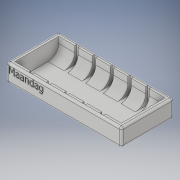
# Autodesk Inventor part: Maandag
Saved by Autodesk Inventor 2019 (Build 230136000, 136)
## iProperties
Created: 2020-10-20
Part Number: Maandag
Material: Generic
Document SubType Name: Modeling
Designer: daanswinters
Density: 1 g/cm^3
Appearance: Default
Author: daanswinters
Autodesk Inventor part; units mm, degrees
ref_plane "YZ Plane" through (0, 0, 0) normal (1, 0, 0) x (0, 1, 0)
ref_plane "XZ Plane" through (0, 0, 0) normal (0, 1, 0) x (-1, 0, 0)
ref_plane "XY Plane" through (0, 0, 0) normal (0, 0, 1) x (1, 0, 0)
sketch "Sketch1" plane through (0, 0, 0) normal (0, 0, 1) x (1, 0, 0)
  line L0 (55, -8.5) -> (-55, -8.5)
  line L1 (-55, -8.5) -> (-55, 8.5)
  line L2 (-55, 8.5) -> (55, 8.5)
  line L3 (55, 8.5) -> (55, -8.5)
  line L4 (55, -8.5) -> (-55, 8.5) construction
  line L5 (-55, -8.5) -> (55, 8.5) construction
  point P0 (0, 0)
  dimension "d0" = 110
  dimension "d1" = 17
  constraints: 12 end point, 2 midpoint, 2 parallel, 1 horizontal, 1 perpendicular
  measures "d0" distance of L1.end L2.end
  measures "d1" distance of L0.end L1.end
extrude "Extrusion1" add sketch "Sketch1" along normal blind 50
sketch "Sketch2" plane through (-55, 8.5, 0) normal (0, 1, 0) x (1, 0, 0)
  line L0 (0, 0) -> (0, -50) projected
  line L1 (110, -50) -> (0, -50)
  line L2 (0, -50) -> (0, 0)
  line L3 (0, 0) -> (110, 0)
  line L4 (110, 0) -> (110, -50)
  line L5 (110, -50) -> (0, 0) construction
  line L6 (0, -50) -> (110, 0) construction
  line L7 (106, -46) -> (106, -4)
  line L8 (4, -4) -> (4, -46)
  line L9 (56.15, -2) -> (53.85, -2)
  line L10 (53.85, -48) -> (56.15, -48)
  line L11 (56.15, -2) -> (53.85, -48) construction
  line L12 (53.85, -2) -> (56.15, -48) construction
  line L13 (73.15, -2) -> (70.85, -2)
  line L14 (70.85, -48) -> (73.15, -48)
  line L15 (73.15, -2) -> (70.85, -48) construction
  line L16 (70.85, -2) -> (73.15, -48) construction
  line L17 (0, -25) -> (110, -25) construction
  line L18 (87.85, -2) -> (90.15, -2)
  line L19 (90.15, -48) -> (87.85, -48)
  line L20 (87.85, -2) -> (90.15, -48) construction
  line L21 (90.15, -2) -> (87.85, -48) construction
  line L22 (36.85, -2) -> (39.15, -2)
  line L23 (39.15, -48) -> (36.85, -48)
  line L24 (36.85, -2) -> (39.15, -48) construction
  line L25 (39.15, -2) -> (36.85, -48) construction
  line L26 (19.85, -2) -> (22.15, -2)
  line L27 (22.15, -48) -> (19.85, -48)
  line L28 (19.85, -2) -> (22.15, -48) construction
  line L29 (22.15, -2) -> (19.85, -48) construction
  line L30 (90.15, -2) -> (90.15, -4)
  line L31 (90.15, -46) -> (90.15, -48)
  line L32 (87.85, -48) -> (87.85, -46)
  line L33 (87.85, -4) -> (87.85, -2)
  line L34 (73.15, -48) -> (73.15, -46)
  line L35 (73.15, -4) -> (73.15, -2)
  line L36 (70.85, -2) -> (70.85, -4)
  line L37 (70.85, -46) -> (70.85, -48)
  line L38 (56.15, -4) -> (56.15, -2)
  line L39 (53.85, -2) -> (53.85, -4)
  line L40 (53.85, -46) -> (53.85, -48)
  line L41 (56.15, -48) -> (56.15, -46)
  line L42 (39.15, -2) -> (39.15, -4)
  line L43 (39.15, -46) -> (39.15, -48)
  line L44 (36.85, -48) -> (36.85, -46)
  line L45 (36.85, -4) -> (36.85, -2)
  line L46 (22.15, -2) -> (22.15, -4)
  line L47 (19.85, -48) -> (19.85, -46)
  line L48 (19.85, -4) -> (19.85, -2)
  line L49 (22.15, -46) -> (22.15, -48)
  line L50 (4, -46) -> (19.95, -46)
  line L51 (22.05, -46) -> (36.95, -46)
  line L52 (39.05, -46) -> (53.95, -46)
  line L53 (56.05, -46) -> (70.95, -46)
  line L54 (73.05, -46) -> (87.95, -46)
  line L55 (90.05, -46) -> (106, -46)
  line L56 (106, -4) -> (90.05, -4)
  line L57 (87.95, -4) -> (73.05, -4)
  line L58 (70.95, -4) -> (56.05, -4)
  line L59 (53.95, -4) -> (39.05, -4)
  line L60 (36.95, -4) -> (22.05, -4)
  line L61 (19.95, -4) -> (4, -4)
  point P0 (55, 0)
  point P1 (55, -25)
  point P2 (72, -25)
  point P3 (89, -25)
  point P4 (38, -25)
  point P5 (21, -25)
  dimension "d4" = 65.556
  dimension "d5" = 110
  dimension "d7" = 2.3
  dimension "d8" = 46
  dimension "d9" = 2.3
  dimension "d10" = 46
  dimension "d11" = 0
  dimension "d12" = 2.3
  dimension "d13" = 46
  dimension "d14" = 2.3
  dimension "d15" = 46
  dimension "d16" = 2.3
  dimension "d17" = 46
  dimension "d18" = 17
  dimension "d19" = 17
  dimension "d20" = 17
  dimension "d21" = 17
  dimension "d22" = 2.862
  dimension "d23" = 2.862
  dimension "d24" = 106
  dimension "d25" = 4
  dimension "d26" = 42
  dimension "d27" = 2
  dimension "d28" = 0
  dimension "d29" = 42
  dimension "d30" = 0
  dimension "d31" = 42
  dimension "d32" = 0
  dimension "d33" = 42
  dimension "d34" = 0
  dimension "d35" = 42
  dimension "d36" = 0
  dimension "d37" = 42
  constraints: 122 end point, 73 parallel, 43 point on line, 17 perpendicular, 14 midpoint, 6 horizontal
  measures "d4" angle of L5 L0
  measures "d5" distance between parallel lines of L4 L0
  measures "d7" distance of L10.end L10.start
  measures "d8" distance of L10.start L9.end
  measures "d9" distance of L14.end L14.start
  measures "d10" distance of L14.start L13.end
  measures "d11" distance from line of L17 point (72, -25)
  measures "d12" distance of L19.start L19.end
  measures "d13" distance of L18.end L19.start
  measures "d14" distance of L23.start L23.end
  measures "d15" distance of L22.end L23.start
  measures "d16" distance of L27.start L27.end
  measures "d17" distance of L26.end L27.start
  measures "d18" distance of point (72, -25) point (55, -25)
  measures "d19" distance of point (89, -25) point (72, -25)
  measures "d20" distance of point (38, -25) point (55, -25)
  measures "d21" distance of point (21, -25) point (38, -25)
  measures "d22" angle of L0 L20
  measures "d23" angle of L0 L21
  measures "d24" distance between parallel lines of L7 L0
  measures "d25" distance between parallel lines of L8 L0
  measures "d26" distance between parallel lines of L56 L55
  measures "d27" distance between parallel lines of L56 L18
  measures "d28" distance between parallel lines of L56 L57
  measures "d29" distance between parallel lines of L56 L54
  measures "d30" distance between parallel lines of L56 L58
  measures "d31" distance between parallel lines of L56 L53
  measures "d32" distance between parallel lines of L56 L59
  measures "d33" distance between parallel lines of L56 L52
  measures "d34" distance between parallel lines of L56 L60
  measures "d35" distance between parallel lines of L56 L51
  measures "d36" distance between parallel lines of L56 L61
  measures "d37" distance between parallel lines of L56 L50
extrude "Extrusion2" cut sketch "Sketch2" against normal blind 16 contours L55 L31 L19 L32 L54 L34 L14 L37 L53 L41 L10 L40 L52 L43 L23 L44 L51 L49 L27 L47 L50 L8 L61 L48 L26 L46 L60 L45 L22 L42 L59 L39 L9 L38 L58 L36 L13 L35 L57 L33 L18 L30 L56 L7
fillet "Fillet1" radius 2 12 edges at (-55, 0, 50) (-55, 0, 0) (55, 0, 50) (55, 0, 0) (0, 8.5, 50) (-55, 8.5, 25) (0, 8.5, 0) (55, 8.5, 25) (55, -8.5, 25) (0, -8.5, 50) (-55, -8.5, 25) (0, -8.5, 0)
fillet "Fillet2" radius 10 6 edges at (-43.075, -7.5, 4) (-25.5, -7.5, 4) (-8.5, -7.5, 4) (8.5, -7.5, 4) (25.5, -7.5, 4) (43.075, -7.5, 4)
sketch "Sketch3" plane through (35.15, 8.5, 4) normal (0, 1, 0) x (1, 0, 0)
  line L0 (-70.3, -44) -> (-70.3, -42) projected
  line L1 (-51, 2) -> (-53.3, 2)
  line L2 (-34, 2) -> (-34, 0) projected
  line L3 (-36.3, -44) -> (-36.3, -42) projected
  line L4 (-19.3, -44) -> (-19.3, -42) projected
  line L5 (-2.3, -44) -> (-2.3, -42) projected
  line L6 (0, 2) -> (0, 0) projected
  line L7 (-19.8, 2) -> (-16.5, 2)
  line L8 (-16.5, 2) -> (-16.5, -44)
  line L9 (-16.5, -44) -> (-19.8, -44)
  line L10 (-19.8, -44) -> (-19.8, 2)
  line L11 (-19.8, 2) -> (-16.5, -44) construction
  line L12 (-16.5, 2) -> (-19.8, -44) construction
  line L13 (-2.8, -44) -> (0.5, -44)
  line L14 (0.5, -44) -> (0.5, 2)
  line L15 (0.5, 2) -> (-2.8, 2)
  line L16 (-2.8, 2) -> (-2.8, -44)
  line L17 (-2.8, -44) -> (0.5, 2) construction
  line L18 (0.5, -44) -> (-2.8, 2) construction
  line L19 (-36.8, -44) -> (-33.5, -44)
  line L20 (-33.5, -44) -> (-33.5, 2)
  line L21 (-33.5, 2) -> (-36.8, 2)
  line L22 (-36.8, 2) -> (-36.8, -44)
  line L23 (-36.8, -44) -> (-33.5, 2) construction
  line L24 (-33.5, -44) -> (-36.8, 2) construction
  line L25 (-51, 2) -> (-36.3, 2) projected
  line L26 (-53.8, -44) -> (-50.5, -44)
  line L27 (-50.5, -44) -> (-50.5, 2)
  line L28 (-50.5, 2) -> (-53.8, 2)
  line L29 (-53.8, 2) -> (-53.8, -44)
  line L30 (-53.8, -44) -> (-50.5, 2) construction
  line L31 (-50.5, -44) -> (-53.8, 2) construction
  line L32 (-53.3, -44) -> (-68, -44) projected
  line L33 (-70.8, 2) -> (-67.5, 2)
  line L34 (-67.5, 2) -> (-67.5, -44)
  line L35 (-67.5, -44) -> (-70.8, -44)
  line L36 (-70.8, -44) -> (-70.8, 2)
  line L37 (-70.8, 2) -> (-67.5, -44) construction
  line L38 (-67.5, 2) -> (-70.8, -44) construction
  point P0 (-35.15, 4)
  point P1 (-68, 2)
  point P2 (-17, 2)
  point P3 (-18.15, -21)
  point P4 (-1.15, -21)
  point P5 (-35.15, -21)
  point P6 (-52.15, -21)
  point P7 (-69.15, -21)
  dimension "d42" = 3.3
  dimension "d43" = 46
  dimension "d44" = 3.3
  dimension "d45" = 3.3
  dimension "d46" = 3.3
  dimension "d47" = 3.3
  dimension "d48" = 90
  dimension "d49" = 0.5
  dimension "d50" = 16.5
  dimension "d51" = 33.5
  dimension "d52" = 50.5
  dimension "d53" = 67.5
  dimension "d54" = 46
  dimension "d55" = 0
  dimension "d56" = 53.3
  constraints: 62 end point, 14 parallel, 10 midpoint, 5 horizontal, 5 perpendicular, 3 point on line
  measures "d42" distance of L8.end L9.end
  measures "d43" distance of L7.end L8.end
  measures "d44" distance of L15.end L14.end
  measures "d45" distance of L21.end L20.end
  measures "d46" distance of L28.end L27.end
  measures "d47" distance of L34.end L35.end
  measures "d48" angle of L6 L1
  measures "d49" distance between parallel lines of L6 L14
  measures "d50" distance between parallel lines of L6 L8
  measures "d51" distance between parallel lines of L6 L20
  measures "d52" distance between parallel lines of L6 L27
  measures "d53" distance between parallel lines of L6 L34
  measures "d54" distance between parallel lines of L25 L9
  measures "d55" distance between parallel lines of L15 L25
  measures "d56" distance from line of L1.end L6
extrude "Extrusion3" cut sketch "Sketch3" against normal blind 16
sketch "Sketch4" plane through (0, 0, 50) normal (0, 0, 1) x (1, 0, 0)
  line L0 (-52.9749, 6.5012) -> (53.0345, 6.5012) construction
  line L1 (53.0345, 6.5012) -> (53.0345, -6.5247) construction
  line L2 (53.0345, -6.5247) -> (-52.9749, -6.5247) construction
  line L3 (-52.9749, -6.5247) -> (-52.9749, 6.5012) construction
  line L4 (-47.127, 0.1294) -> (-47.9377, 0.1294)
  line L5 (-47.9377, 0.1294) -> (-47.9377, 5.3841)
  line L6 (-47.9377, 5.3841) -> (-49.5295, 1.8101)
  line L7 (-49.5295, 1.8101) -> (-50.0238, 1.8101)
  line L8 (-50.0238, 1.8101) -> (-51.6007, 5.3841)
  line L9 (-51.6007, 5.3841) -> (-51.6007, 0.1294)
  line L10 (-51.6007, 0.1294) -> (-52.357, 0.1294)
  line L11 (-52.357, 0.1294) -> (-52.357, 6.2294)
  line L12 (-52.357, 6.2294) -> (-51.2497, 6.2294)
  line L13 (-51.2497, 6.2294) -> (-49.7272, 2.8333)
  line L14 (-49.7272, 2.8333) -> (-48.2541, 6.2294)
  line L15 (-48.2541, 6.2294) -> (-47.127, 6.2294)
  line L16 (-47.127, 6.2294) -> (-47.127, 0.1294)
  spline S0 degree 2 poles (-43.3998, 0.6138) (-43.4937, 0.5446) (-43.8101, 0.2974) (-43.9584, 0.2233) knots 0 0 0 1 2 2 2
  spline S1 degree 2 poles (-43.9584, 0.2233) (-44.1611, 0.1145) (-44.5417, 0.0008) (-44.8877, 0.0008) knots 0 0 0 1 2 2 2
  spline S2 degree 2 poles (-44.8877, 0.0008) (-45.1695, 0.0008) (-45.6787, 0.2134) (-45.8714, 0.4062) knots 0 0 0 1 2 2 2
  spline S3 degree 2 poles (-45.8714, 0.4062) (-46.0543, 0.594) (-46.2768, 1.1477) (-46.2768, 1.4542) knots 0 0 0 1 2 2 2
  spline S4 degree 2 poles (-46.2768, 1.4542) (-46.2768, 1.9287) (-45.8764, 2.601) (-45.4414, 2.7938) knots 0 0 0 1 2 2 2
  spline S5 degree 2 poles (-45.4414, 2.7938) (-45.0558, 2.9718) (-44.0078, 3.1052) (-43.3998, 3.1398) knots 0 0 0 1 2 2 2
  line L17 (-43.3998, 3.1398) -> (-43.3998, 3.2881)
  spline S6 degree 2 poles (-43.3998, 3.2881) (-43.3998, 3.5551) (-43.5629, 3.8863) (-43.7112, 3.9802) knots 0 0 0 1 2 2 2
  spline S7 degree 2 poles (-43.7112, 3.9802) (-43.8595, 4.0741) (-44.2847, 4.1334) (-44.512, 4.1334) knots 0 0 0 1 2 2 2
  spline S8 degree 2 poles (-44.512, 4.1334) (-44.779, 4.1334) (-45.5007, 3.9752) (-45.8616, 3.822) knots 0 0 0 1 2 2 2
  line L18 (-45.8616, 3.822) -> (-45.906, 3.822)
  line L19 (-45.906, 3.822) -> (-45.906, 4.608)
  spline S9 degree 2 poles (-45.906, 4.608) (-45.6935, 4.6673) (-44.8976, 4.8156) (-44.5071, 4.8156) knots 0 0 0 1 2 2 2
  spline S10 degree 2 poles (-44.5071, 4.8156) (-44.0325, 4.8156) (-43.385, 4.6673) (-43.1279, 4.4745) knots 0 0 0 1 2 2 2
  spline S11 degree 2 poles (-43.1279, 4.4745) (-42.8758, 4.2867) (-42.6287, 3.6885) (-42.6287, 3.2585) knots 0 0 0 1 2 2 2
  line L20 (-42.6287, 3.2585) -> (-42.6287, 0.1294)
  line L21 (-42.6287, 0.1294) -> (-43.3998, 0.1294)
  line L22 (-43.3998, 0.1294) -> (-43.3998, 0.6138)
  line L23 (-43.3998, 1.2564) -> (-43.3998, 2.5269)
  spline S12 degree 2 poles (-43.3998, 2.5269) (-43.6766, 2.5021) (-44.512, 2.4181) (-44.774, 2.339) knots 0 0 0 1 2 2 2
  spline S13 degree 2 poles (-44.774, 2.339) (-45.0805, 2.2451) (-45.4809, 1.8546) (-45.4809, 1.5085) knots 0 0 0 1 2 2 2
  spline S14 degree 2 poles (-45.4809, 1.5085) (-45.4809, 1.1131) (-45.036, 0.7127) (-44.6109, 0.7127) knots 0 0 0 1 2 2 2
  spline S15 degree 2 poles (-44.6109, 0.7127) (-44.25, 0.7127) (-43.6569, 1.0241) (-43.3998, 1.2564) knots 0 0 0 1 2 2 2
  spline S16 degree 2 poles (-38.9953, 0.6138) (-39.0893, 0.5446) (-39.4056, 0.2974) (-39.5539, 0.2233) knots 0 0 0 1 2 2 2
  spline S17 degree 2 poles (-39.5539, 0.2233) (-39.7566, 0.1145) (-40.1372, 0.0008) (-40.4833, 0.0008) knots 0 0 0 1 2 2 2
  spline S18 degree 2 poles (-40.4833, 0.0008) (-40.765, 0.0008) (-41.2742, 0.2134) (-41.467, 0.4062) knots 0 0 0 1 2 2 2
  spline S19 degree 2 poles (-41.467, 0.4062) (-41.6499, 0.594) (-41.8723, 1.1477) (-41.8723, 1.4542) knots 0 0 0 1 2 2 2
  spline S20 degree 2 poles (-41.8723, 1.4542) (-41.8723, 1.9287) (-41.4719, 2.601) (-41.0369, 2.7938) knots 0 0 0 1 2 2 2
  spline S21 degree 2 poles (-41.0369, 2.7938) (-40.6513, 2.9718) (-39.6034, 3.1052) (-38.9953, 3.1398) knots 0 0 0 1 2 2 2
  line L24 (-38.9953, 3.1398) -> (-38.9953, 3.2881)
  spline S22 degree 2 poles (-38.9953, 3.2881) (-38.9953, 3.5551) (-39.1585, 3.8863) (-39.3068, 3.9802) knots 0 0 0 1 2 2 2
  spline S23 degree 2 poles (-39.3068, 3.9802) (-39.4551, 4.0741) (-39.8802, 4.1334) (-40.1076, 4.1334) knots 0 0 0 1 2 2 2
  spline S24 degree 2 poles (-40.1076, 4.1334) (-40.3745, 4.1334) (-41.0962, 3.9752) (-41.4571, 3.822) knots 0 0 0 1 2 2 2
  line L25 (-41.4571, 3.822) -> (-41.5016, 3.822)
  line L26 (-41.5016, 3.822) -> (-41.5016, 4.608)
  spline S25 degree 2 poles (-41.5016, 4.608) (-41.289, 4.6673) (-40.4932, 4.8156) (-40.1026, 4.8156) knots 0 0 0 1 2 2 2
  spline S26 degree 2 poles (-40.1026, 4.8156) (-39.6281, 4.8156) (-38.9805, 4.6673) (-38.7235, 4.4745) knots 0 0 0 1 2 2 2
  spline S27 degree 2 poles (-38.7235, 4.4745) (-38.4714, 4.2867) (-38.2242, 3.6885) (-38.2242, 3.2585) knots 0 0 0 1 2 2 2
  line L27 (-38.2242, 3.2585) -> (-38.2242, 0.1294)
  line L28 (-38.2242, 0.1294) -> (-38.9953, 0.1294)
  line L29 (-38.9953, 0.1294) -> (-38.9953, 0.6138)
  line L30 (-38.9953, 1.2564) -> (-38.9953, 2.5269)
  spline S28 degree 2 poles (-38.9953, 2.5269) (-39.2722, 2.5021) (-40.1076, 2.4181) (-40.3696, 2.339) knots 0 0 0 1 2 2 2
  spline S29 degree 2 poles (-40.3696, 2.339) (-40.6761, 2.2451) (-41.0765, 1.8546) (-41.0765, 1.5085) knots 0 0 0 1 2 2 2
  spline S30 degree 2 poles (-41.0765, 1.5085) (-41.0765, 1.1131) (-40.6316, 0.7127) (-40.2064, 0.7127) knots 0 0 0 1 2 2 2
  spline S31 degree 2 poles (-40.2064, 0.7127) (-39.8456, 0.7127) (-39.2524, 1.0241) (-38.9953, 1.2564) knots 0 0 0 1 2 2 2
  line L31 (-33.5479, 0.1294) -> (-34.319, 0.1294)
  line L32 (-34.319, 0.1294) -> (-34.319, 2.7394)
  spline S32 degree 2 poles (-34.319, 2.7394) (-34.319, 3.0558) (-34.3783, 3.5995) (-34.4673, 3.7627) knots 0 0 0 1 2 2 2
  spline S33 degree 2 poles (-34.4673, 3.7627) (-34.5612, 3.9357) (-34.8974, 4.1038) (-35.1841, 4.1038) knots 0 0 0 1 2 2 2
  spline S34 degree 2 poles (-35.1841, 4.1038) (-35.4708, 4.1038) (-36.0788, 3.7973) (-36.3705, 3.5501) knots 0 0 0 1 2 2 2
  line L33 (-36.3705, 3.5501) -> (-36.3705, 0.1294)
  line L34 (-36.3705, 0.1294) -> (-37.1416, 0.1294)
  line L35 (-37.1416, 0.1294) -> (-37.1416, 4.7068)
  line L36 (-37.1416, 4.7068) -> (-36.3705, 4.7068)
  line L37 (-36.3705, 4.7068) -> (-36.3705, 4.1977)
  spline S35 degree 2 poles (-36.3705, 4.1977) (-36.0244, 4.5091) (-35.3571, 4.8354) (-34.9814, 4.8354) knots 0 0 0 1 2 2 2
  spline S36 degree 2 poles (-34.9814, 4.8354) (-34.3091, 4.8354) (-33.5479, 3.9456) (-33.5479, 3.1003) knots 0 0 0 1 2 2 2
  line L38 (-33.5479, 3.1003) -> (-33.5479, 0.1294)
  line L39 (-28.9457, 0.1294) -> (-29.7168, 0.1294)
  line L40 (-29.7168, 0.1294) -> (-29.7168, 0.594)
  spline S37 degree 2 poles (-29.7168, 0.594) (-29.8948, 0.4457) (-30.1568, 0.248) (-30.3347, 0.164) knots 0 0 0 1 2 2 2
  spline S38 degree 2 poles (-30.3347, 0.164) (-30.4979, 0.0849) (-30.8488, 0.0008) (-31.0812, 0.0008) knots 0 0 0 1 2 2 2
  spline S39 degree 2 poles (-31.0812, 0.0008) (-31.4569, 0.0008) (-32.0896, 0.3123) (-32.312, 0.6138) knots 0 0 0 1 2 2 2
  spline S40 degree 2 poles (-32.312, 0.6138) (-32.5345, 0.9153) (-32.7817, 1.8051) (-32.7817, 2.3835) knots 0 0 0 1 2 2 2
  spline S41 degree 2 poles (-32.7817, 2.3835) (-32.7817, 2.9866) (-32.4702, 3.8665) (-32.1983, 4.1977) knots 0 0 0 1 2 2 2
  spline S42 degree 2 poles (-32.1983, 4.1977) (-31.9462, 4.4943) (-31.2394, 4.8354) (-30.8488, 4.8354) knots 0 0 0 1 2 2 2
  spline S43 degree 2 poles (-30.8488, 4.8354) (-30.5077, 4.8354) (-29.9986, 4.6821) (-29.7168, 4.5239) knots 0 0 0 1 2 2 2
  line L41 (-29.7168, 4.5239) -> (-29.7168, 6.5012)
  line L42 (-29.7168, 6.5012) -> (-28.9457, 6.5012)
  line L43 (-28.9457, 6.5012) -> (-28.9457, 0.1294)
  line L44 (-29.7168, 1.2416) -> (-29.7168, 3.8863)
  spline S44 degree 2 poles (-29.7168, 3.8863) (-30.0035, 4.0247) (-30.4583, 4.1285) (-30.7203, 4.1285) knots 0 0 0 1 2 2 2
  spline S45 degree 2 poles (-30.7203, 4.1285) (-31.3135, 4.1285) (-31.9858, 3.2387) (-31.9858, 2.3983) knots 0 0 0 1 2 2 2
  spline S46 degree 2 poles (-31.9858, 2.3983) (-31.9858, 1.5876) (-31.4717, 0.7324) (-30.9032, 0.7324) knots 0 0 0 1 2 2 2
  spline S47 degree 2 poles (-30.9032, 0.7324) (-30.6017, 0.7324) (-29.9887, 1.0093) (-29.7168, 1.2416) knots 0 0 0 1 2 2 2
  spline S48 degree 2 poles (-25.2778, 0.6138) (-25.3717, 0.5446) (-25.6881, 0.2974) (-25.8364, 0.2233) knots 0 0 0 1 2 2 2
  spline S49 degree 2 poles (-25.8364, 0.2233) (-26.039, 0.1145) (-26.4197, 0.0008) (-26.7657, 0.0008) knots 0 0 0 1 2 2 2
  spline S50 degree 2 poles (-26.7657, 0.0008) (-27.0475, 0.0008) (-27.5566, 0.2134) (-27.7494, 0.4062) knots 0 0 0 1 2 2 2
  spline S51 degree 2 poles (-27.7494, 0.4062) (-27.9323, 0.594) (-28.1547, 1.1477) (-28.1547, 1.4542) knots 0 0 0 1 2 2 2
  spline S52 degree 2 poles (-28.1547, 1.4542) (-28.1547, 1.9287) (-27.7543, 2.601) (-27.3193, 2.7938) knots 0 0 0 1 2 2 2
  spline S53 degree 2 poles (-27.3193, 2.7938) (-26.9338, 2.9718) (-25.8858, 3.1052) (-25.2778, 3.1398) knots 0 0 0 1 2 2 2
  line L45 (-25.2778, 3.1398) -> (-25.2778, 3.2881)
  spline S54 degree 2 poles (-25.2778, 3.2881) (-25.2778, 3.5551) (-25.4409, 3.8863) (-25.5892, 3.9802) knots 0 0 0 1 2 2 2
  spline S55 degree 2 poles (-25.5892, 3.9802) (-25.7375, 4.0741) (-26.1626, 4.1334) (-26.39, 4.1334) knots 0 0 0 1 2 2 2
  spline S56 degree 2 poles (-26.39, 4.1334) (-26.6569, 4.1334) (-27.3787, 3.9752) (-27.7395, 3.822) knots 0 0 0 1 2 2 2
  line L46 (-27.7395, 3.822) -> (-27.784, 3.822)
  line L47 (-27.784, 3.822) -> (-27.784, 4.608)
  spline S57 degree 2 poles (-27.784, 4.608) (-27.5714, 4.6673) (-26.7756, 4.8156) (-26.3851, 4.8156) knots 0 0 0 1 2 2 2
  spline S58 degree 2 poles (-26.3851, 4.8156) (-25.9105, 4.8156) (-25.2629, 4.6673) (-25.0059, 4.4745) knots 0 0 0 1 2 2 2
  spline S59 degree 2 poles (-25.0059, 4.4745) (-24.7538, 4.2867) (-24.5066, 3.6885) (-24.5066, 3.2585) knots 0 0 0 1 2 2 2
  line L48 (-24.5066, 3.2585) -> (-24.5066, 0.1294)
  line L49 (-24.5066, 0.1294) -> (-25.2778, 0.1294)
  line L50 (-25.2778, 0.1294) -> (-25.2778, 0.6138)
  line L51 (-25.2778, 1.2564) -> (-25.2778, 2.5269)
  spline S60 degree 2 poles (-25.2778, 2.5269) (-25.5546, 2.5021) (-26.39, 2.4181) (-26.652, 2.339) knots 0 0 0 1 2 2 2
  spline S61 degree 2 poles (-26.652, 2.339) (-26.9585, 2.2451) (-27.3589, 1.8546) (-27.3589, 1.5085) knots 0 0 0 1 2 2 2
  spline S62 degree 2 poles (-27.3589, 1.5085) (-27.3589, 1.1131) (-26.914, 0.7127) (-26.4889, 0.7127) knots 0 0 0 1 2 2 2
  spline S63 degree 2 poles (-26.4889, 0.7127) (-26.128, 0.7127) (-25.5348, 1.0241) (-25.2778, 1.2564) knots 0 0 0 1 2 2 2
  spline S64 degree 2 poles (-23.2609, -0.6022) (-23.1818, -0.6368) (-22.8803, -0.7456) (-22.6875, -0.7901) knots 0 0 0 1 2 2 2
  spline S65 degree 2 poles (-22.6875, -0.7901) (-22.4749, -0.8445) (-22.1141, -0.9087) (-21.9015, -0.9087) knots 0 0 0 1 2 2 2
  spline S66 degree 2 poles (-21.9015, -0.9087) (-21.5456, -0.9087) (-21.0513, -0.7209) (-20.9129, -0.5528) knots 0 0 0 1 2 2 2
  spline S67 degree 2 poles (-20.9129, -0.5528) (-20.7794, -0.3847) (-20.6756, 0.0552) (-20.6756, 0.337) knots 0 0 0 1 2 2 2
  line L52 (-20.6756, 0.337) -> (-20.6756, 0.7374)
  spline S68 degree 2 poles (-20.6756, 0.7374) (-20.987, 0.4655) (-21.5851, 0.2085) (-22.035, 0.2085) knots 0 0 0 1 2 2 2
  spline S69 degree 2 poles (-22.035, 0.2085) (-22.816, 0.2085) (-23.7404, 1.3701) (-23.7404, 2.4626) knots 0 0 0 1 2 2 2
  spline S70 degree 2 poles (-23.7404, 2.4626) (-23.7404, 3.0311) (-23.4191, 3.911) (-23.1522, 4.2224) knots 0 0 0 1 2 2 2
  spline S71 degree 2 poles (-23.1522, 4.2224) (-22.8951, 4.5141) (-22.1882, 4.8354) (-21.8125, 4.8354) knots 0 0 0 1 2 2 2
  spline S72 degree 2 poles (-21.8125, 4.8354) (-21.4566, 4.8354) (-20.9376, 4.6673) (-20.6756, 4.5141) knots 0 0 0 1 2 2 2
  line L53 (-20.6756, 4.5141) -> (-20.6311, 4.7068)
  line L54 (-20.6311, 4.7068) -> (-19.9044, 4.7068)
  line L55 (-19.9044, 4.7068) -> (-19.9044, 0.6534)
  spline S73 degree 2 poles (-19.9044, 0.6534) (-19.9044, -0.5133) (-20.9178, -1.6008) (-21.9608, -1.6008) knots 0 0 0 1 2 2 2
  spline S74 degree 2 poles (-21.9608, -1.6008) (-22.297, -1.6008) (-22.9989, -1.492) (-23.3005, -1.403) knots 0 0 0 1 2 2 2
  line L56 (-23.3005, -1.403) -> (-23.3005, -0.6022)
  line L57 (-23.3005, -0.6022) -> (-23.2609, -0.6022)
  line L58 (-20.6756, 1.3701) -> (-20.6756, 3.8863)
  spline S75 degree 2 poles (-20.6756, 3.8863) (-20.9623, 4.0247) (-21.4467, 4.1433) (-21.6889, 4.1433) knots 0 0 0 1 2 2 2
  spline S76 degree 2 poles (-21.6889, 4.1433) (-22.2723, 4.1433) (-22.9445, 3.2832) (-22.9445, 2.4774) knots 0 0 0 1 2 2 2
  spline S77 degree 2 poles (-22.9445, 2.4774) (-22.9445, 1.7162) (-22.4354, 0.9203) (-21.862, 0.9203) knots 0 0 0 1 2 2 2
  spline S78 degree 2 poles (-21.862, 0.9203) (-21.5604, 0.9203) (-20.9277, 1.1576) (-20.6756, 1.3701) knots 0 0 0 1 2 2 2
  point P0 (0, 0)
  constraints: 2 other
extrude "Extrusion4" cut sketch "Sketch4" against normal blind 0.5
fillet "Fillet3" radius 10 6 edges at (-43.325, -7.5, 46) (-25.5, -7.5, 46) (-8.5, -7.5, 46) (8.5, -7.5, 46) (25.5, -7.5, 46) (43.325, -7.5, 46)
body "Solid1"
